# Autodesk Inventor part: m1.5_bolt_12mm
Saved by Autodesk Inventor 2021 (Build 250183000, 183)
## iProperties
Created: 2021-03-15
Part Number: m1.5_bolt_12mm
Material: Brass, Soft Yellow
Document SubType Name: Modeling
Designer: Tomasz Lisowski
Density: 8.47 g/cm^3
Appearance: Brass - Satin
Author: Tomasz Lisowski
Autodesk Inventor part; units mm, degrees
ref_plane "YZ Plane" through (0, 0, 0) normal (1, 0, 0) x (0, 1, 0)
ref_plane "XZ Plane" through (0, 0, 0) normal (0, 1, 0) x (-1, 0, 0)
ref_plane "XY Plane" through (0, 0, 0) normal (0, 0, 1) x (1, 0, 0)
sketch "Sketch1" plane through (0, 0, 0) normal (0, 1, 0) x (-1, 0, 0)
  circle A0 centre (0, 0) radius 1.5
  dimension "d0" = 3
  constraints: 1 centre point, 1 coincident
  measures "d0" diameter of A0
extrude "Extrusion1" add sketch "Sketch1" along normal blind 1
sketch "Sketch2" plane through (0, 1, 0) normal (0, 1, 0) x (1, 0, 0)
  circle A0 centre (0, 0) radius 0.75
  dimension "d3" = 1.5
  constraints: 1 centre point, 1 coincident
  measures "d3" diameter of A0
extrude "Extrusion2" add sketch "Sketch2" along normal blind 12
sketch "Sketch3" plane through (0, 0, 0) normal (0, -1, 0) x (1, 0, 0)
  line L0 (0.25, 1.5) -> (-0.25, 1.5)
  line L1 (-0.25, 1.5) -> (-0.25, -1.5)
  line L2 (-0.25, -1.5) -> (0.25, -1.5)
  line L3 (0.25, -1.5) -> (0.25, 1.5)
  line L4 (0.25, 1.5) -> (-0.25, -1.5) construction
  line L5 (-0.25, 1.5) -> (0.25, -1.5) construction
  circle A0 centre (0, 0) radius 1.5 projected
  point P0 (0.25, -1.479)
  point P1 (0.25, 1.479)
  point P2 (-0.25, 1.479)
  point P3 (-0.25, -1.479)
  dimension "d6" = 0.5
  constraints: 12 end point, 2 midpoint, 2 parallel, 1 horizontal, 1 perpendicular, 1 tangent
  measures "d6" distance of L2.end L1.end
extrude "Extrusion3" cut sketch "Sketch3" against normal blind 0.3 contours A0 L3 L1
body "Solid1"
